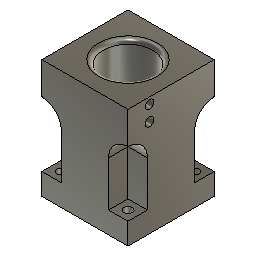
endstop new Z sls v2 (Autodesk Fusion 360 design; units mm, degrees)
Autodesk Fusion 360 part; units mm, degrees
sketch "Skizze1" plane through (0, 0, 0) normal (0, 0, 1) x (1, 0, 0)
  line L0 (4.5, 4.5) -> (35.5, 4.5)
  line L1 (35.5, 4.5) -> (35.5, 35.5)
  line L2 (35.5, 35.5) -> (4.5, 35.5)
  line L3 (4.5, 35.5) -> (4.5, 4.5)
  line L4 (4.5, 4.5) -> (35.5, 35.5) construction
  line L5 (35.5, 4.5) -> (4.5, 35.5) construction
  circle A0 centre (20, 20) radius 11.5
  circle A1 centre (4.5, 35.5) radius 2
  circle A2 centre (35.5, 35.5) radius 2
  circle A3 centre (4.5, 4.5) radius 2
  circle A4 centre (35.5, 4.5) radius 2
  line L6 (0, 40) -> (40, 40)
  line L7 (40, 40) -> (40, 0)
  line L8 (40, 0) -> (0, 0)
  line L9 (0, 0) -> (0, 40)
  line L10 (0, 40) -> (40, 0) construction
  line L11 (40, 40) -> (0, 0) construction
  point P0 (20, 20)
  point P1 (20, 20)
  dimension "d1" = 31
  dimension "d2" = 31
  dimension "d3" = 23
  dimension "d4" = 4
  dimension "d5" = 4
  dimension "d6" = 4
  dimension "d7" = 4
  dimension "d8" = 40
  dimension "d9" = 40
  constraint horizontal L0
  constraint perpendicular L0 L1
  constraint parallel L0 L2
  constraint parallel L1 L3
  constraint coincident L4 P1
  constraint coincident L5 P1
  constraint coincident P1 P0
  constraint coincident L2.end L3.start
  constraint coincident L1.end L2.start
  constraint coincident L0.start L3.end
  constraint coincident L0.end L1.start
  constraint horizontal L6
  constraint perpendicular L6 L7
  constraint parallel L6 L8
  constraint parallel L7 L9
  constraint coincident L10 P1
  constraint coincident L11 P1
  constraint coincident L8.end L9.start
  measures "d1" distance of L1.end L2.end
  measures "d2" distance of L0.end L1.end
  measures "d3" diameter of A0
  measures "d4" diameter of A1
  measures "d5" diameter of A2
  measures "d6" diameter of A3
  measures "d7" diameter of A4
  measures "d8" distance of L7.end L8.end
  measures "d9" distance of L6.end L7.end
extrude "Extrusion1" add sketch "Skizze1" along normal blind 10 contours L0 L1 L2 L3 A1 A2 A3 A4 | L6 L7 L8 L9
sketch "Skizze2" plane through (0, 0, 10) normal (0, 0, 1) x (-1, 0, 0)
  circle A0 centre (-4.5, -4.5) radius 2
  circle A1 centre (-35.5, -35.5) radius 2
  circle A2 centre (-35.5, -4.5) radius 2
  circle A3 centre (-20, -20) radius 11.5
  circle A4 centre (-4.5, -35.5) radius 2
  line L0 (0, 0) -> (-40, 0)
  line L1 (-40, 0) -> (-40, -40)
  line L2 (-40, -40) -> (0, -40)
  line L3 (0, -40) -> (0, 0)
  line L4 (0, -31) -> (-40, -31)
  line L5 (-40, -31) -> (-40, -9)
  line L6 (-40, -9) -> (0, -9)
  line L7 (0, -9) -> (0, -31)
  line L8 (0, -31) -> (-40, -9) construction
  line L9 (-40, -31) -> (0, -9) construction
  line L10 (-9, -40) -> (-31, -40)
  line L11 (-31, -40) -> (-31, 0)
  line L12 (-31, 0) -> (-9, 0)
  line L13 (-9, 0) -> (-9, -40)
  line L14 (-9, -40) -> (-31, 0) construction
  line L15 (-31, -40) -> (-9, 0) construction
  point P0 (-20, -20)
  point P1 (-20, -20)
  constraint horizontal L4
  constraint perpendicular L4 L5
  constraint parallel L4 L6
  constraint parallel L5 L7
  constraint coincident L8 P1
  constraint coincident L9 P1
  constraint coincident L3 L4.start
  constraint coincident P1 P0
  constraint horizontal L10
  constraint perpendicular L10 L11
  constraint parallel L10 L12
  constraint parallel L11 L13
  constraint coincident L14 P1
  constraint coincident L15 P1
  constraint coincident L2 L10.start
extrude "Extrusion2" add sketch "Skizze2" along normal blind 30 contours A3 L3 L4 L6 L7 L13 | A3 L6 L13 | A3 L4 L13 | A3 L0 L6 L11 L12 L13 | A3 L2 L4 L10 L11 L13 | A3 L6 L11 | A3 L4 L11 | A3 L1 L4 L5 L6 L11
sketch "Skizze3" plane through (0, 0, 40) normal (0, 0, 1) x (-1, 0, 0)
  circle A0 centre (-20, -20) radius 11.5
  line L0 (-9, 0) -> (-31, 0)
  line L1 (-31, 0) -> (-31, -9)
  line L2 (-31, -9) -> (-40, -9)
  line L3 (-40, -9) -> (-40, -31)
  line L4 (-40, -31) -> (-31, -31)
  line L5 (-31, -31) -> (-31, -40)
  line L6 (-31, -40) -> (-9, -40)
  line L7 (-9, -40) -> (-9, -31)
  line L8 (-9, -31) -> (0, -31)
  line L9 (0, -31) -> (0, -9)
  line L10 (0, -9) -> (-9, -9)
  line L11 (-9, -9) -> (-9, 0)
  line L12 (0, -40) -> (-40, -40)
  line L13 (-40, -40) -> (-40, 0)
  line L14 (-40, 0) -> (0, 0)
  line L15 (0, 0) -> (0, -40)
  line L16 (0, -40) -> (-40, 0) construction
  line L17 (-40, -40) -> (0, 0) construction
  point P0 (-20, -20)
  constraint horizontal L12
  constraint perpendicular L12 L13
  constraint parallel L12 L14
  constraint parallel L13 L15
  constraint coincident L16 P0
  constraint coincident L17 P0
  constraint coincident P0 A0.centre
extrude "Extrusion3" add sketch "Skizze3" along normal blind 2
extrude "Extrusion4" add 1 faces at (19.7135, 37.1559, 42) along direction (0, 0, 1) blind 13
sketch "Skizze4" plane through (40, 0, 0) normal (1, 0, 0) x (0, 1, 0)
  line L0 (0, 0) -> (40, 0)
  line L1 (40, 0) -> (40, 10)
  line L2 (40, 10) -> (31, 10)
  line L3 (31, 10) -> (31, 40)
  line L4 (31, 40) -> (40, 40)
  line L5 (40, 40) -> (40, 55)
  line L6 (40, 55) -> (0, 55)
  line L7 (0, 55) -> (0, 40)
  line L8 (0, 40) -> (9, 40)
  line L9 (9, 40) -> (9, 10)
  line L10 (9, 10) -> (0, 10)
  line L11 (0, 10) -> (0, 0)
  circle A0 centre (10, 52) radius 2
  circle A1 centre (10, 45) radius 2
  line L12 (10, 52) -> (10, 45)
  dimension "d18" = 4
  dimension "d19" = 4
  dimension "d26" = 7
  constraint coincident A0.centre L12.start
  constraint perpendicular L6 L12
  constraint coincident A1.centre L12.end
  measures "d18" diameter of A0
  measures "d19" diameter of A1
  measures "d26" distance of A0.centre A1.centre
extrude "Extrusion5" cut sketch "Skizze4" against normal blind 10 contours A0 | A1
fillet "Abrundung1" radius 9 8 edges at (31, 35.5, 40) (35.5, 31, 40) (31, 4.5, 40) (35.5, 9, 40) (4.5, 9, 40) (9, 4.5, 40) (9, 35.5, 40) (4.5, 31, 40)
fillet "Abrundung2" radius 2 1 edges at (30.7218, 15.8414, 55)
